Autodesk Inventor part; units mm, degrees
(part 2 of 2)
ref_plane "to_L_Winkel_1_YZ" through (-98.75, 0, -61.025) normal (0, 0, -1) x (0, -1, 0)
ref_plane "to_L_Winkel_1_ZX" through (-98.75, 0, -61.025) normal (0, -1, 0) x (-1, 0, 0)
ref_plane "to_MP_XY" through (0, 0, -61.125) normal (0, 0, -1) x (1, 0, 0)
ref_plane "to_MP_YZ" through (0, 0, -61.125) normal (1, 0, 0) x (0, -1, 0)
ref_plane "to_MP_ZX" through (0, 0, -61.125) normal (0, -1, 0) x (0, 0, -1)
sketch "Sketch45" plane through (-100, 150, 53.1072) normal (0, 1, 0) x (1, 0, 0)
  circle A0 centre (25, 25) radius 12.5
  line L0 (200, 0) -> (0, 0) projected
  point P0 (100, 53.1072)
  dimension "d92" = 25
  dimension "d93" = 75
  dimension "d94" = 25
  constraints: 1 centre point
  measures "d92" diameter of A0
  measures "d93" horizontal distance of point (100, 53.107) A0.centre
  measures "d94" distance from line of L0 A0.centre
extrude "Extrusion21" cut sketch "Sketch45" against normal blind 10
body "Solid1"
